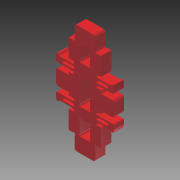
# Autodesk Inventor part: gantry7
Saved by Autodesk Inventor 2012 SP1 (Build 160190100, 190)
## iProperties
Created: 2011-10-14
Part Number: gantry7
Document SubType Name: Modeling
Designer: cramera
Density: 0.952 g/cm^3
Material: High Density Polyethylene
Mass: 48.8041 g
Surface Area: 201.117 cm^2
Volume: 51.2648 cm^3
Autodesk Inventor part; units mm, degrees
ref_plane "YZ Plane" through (0, 0, 0) normal (1, 0, 0) x (0, 1, 0)
ref_plane "XZ Plane" through (0, 0, 0) normal (0, 1, 0) x (-1, 0, 0)
ref_plane "XY Plane" through (0, 0, 0) normal (0, 0, 1) x (1, 0, 0)
derived "skeleton.ipt"
sketch "STOCK_12MM" plane through (0, 0, 0) normal (0, 0, 1) x (1, 0, 0)
  line L0 (457.2, 0) -> (914.4, 0)
  line L1 (914.4, 0) -> (914.4, 914.4)
  line L2 (914.4, 914.4) -> (457.2, 914.4)
  line L3 (457.2, 914.4) -> (457.2, 0)
  line L4 (0, 0) -> (457.2, 0)
  line L5 (457.2, 0) -> (457.2, 914.4)
  line L6 (457.2, 914.4) -> (0, 914.4)
  line L7 (0, 914.4) -> (0, 0)
  constraints: 16 end point
sketch "THROUGH-CUT" plane through (0, 0, 0) normal (0, 0, 1) x (1, 0, 0)
  arc A0 (280.404, 284.8782) -> (278.1589, 282.6331) centre (279.2814, 283.7556) ccw
  line L0 (278.1589, 282.6331) -> (278.1589, 255.1192)
  arc A1 (278.1589, 255.1192) -> (278.1589, 252.8742) centre (279.2814, 253.9967) ccw
  arc A2 (278.1589, 252.8742) -> (280.404, 252.8742) centre (279.2814, 253.9967) ccw
  line L1 (280.404, 252.8742) -> (288.2328, 252.8742)
  arc A3 (288.2328, 252.8742) -> (290.4779, 252.8742) centre (289.3554, 253.9967) ccw
  arc A4 (290.4779, 252.8742) -> (290.4779, 255.1192) centre (289.3554, 253.9967) ccw
  arc A5 (265.0779, 260.9387) -> (262.8328, 260.9387) centre (263.9554, 259.8161) ccw
  arc A6 (265.0779, 258.6936) -> (265.0779, 260.9387) centre (263.9554, 259.8161) ccw
  line L2 (265.0779, 258.6936) -> (265.0779, 257.6367)
  line L3 (265.0779, 257.6367) -> (269.8404, 257.6367)
  arc A7 (271.4279, 256.0492) -> (269.8404, 257.6367) centre (269.8404, 256.0492) ccw
  line L4 (271.4279, 256.0492) -> (271.4279, 255.9222)
  arc A8 (269.8404, 254.3347) -> (271.4279, 255.9222) centre (269.8404, 255.9222) ccw
  line L5 (269.8404, 254.3347) -> (265.0779, 254.3347)
  line L6 (265.0779, 254.3347) -> (251.4254, 254.3347)
  arc A9 (251.4254, 254.3347) -> (249.8379, 252.7494) centre (251.4254, 252.7472) ccw
  line L7 (249.8379, 252.7494) -> (249.8379, 249.0442)
  line L8 (249.8379, 249.0442) -> (250.66, 245.4447)
  line L9 (250.66, 245.4447) -> (252.3779, 245.4447)
  line L10 (252.3779, 245.4447) -> (253.6479, 246.9687)
  line L11 (253.6479, 246.9687) -> (256.2752, 246.9687)
  line L12 (256.2752, 246.9687) -> (265.0779, 246.9687)
  line L13 (265.0779, 246.9687) -> (269.8404, 246.9687)
  arc A10 (271.4279, 245.3812) -> (269.8404, 246.9687) centre (269.8404, 245.3812) ccw
  line L14 (271.4279, 245.3812) -> (271.4279, 245.2542)
  arc A11 (269.8404, 243.6667) -> (271.4279, 245.2542) centre (269.8404, 245.2542) ccw
  line L15 (269.8404, 243.6667) -> (265.0779, 243.6667)
  line L16 (265.0779, 243.6667) -> (265.0779, 222.2037)
  line L17 (265.0779, 222.2037) -> (269.8813, 222.2037)
  arc A12 (272.1264, 222.2037) -> (269.8813, 222.2037) centre (271.0039, 221.0811) ccw
  arc A13 (272.1264, 219.9586) -> (272.1264, 222.2037) centre (271.0039, 221.0811) ccw
  line L18 (272.1264, 219.9586) -> (272.1264, 206.3287)
  line L19 (272.1264, 206.3287) -> (273.7139, 204.7412)
  line L20 (273.7139, 204.7412) -> (294.9229, 204.7412)
  line L21 (294.9229, 204.7412) -> (296.5104, 206.3287)
  line L22 (296.5104, 206.3287) -> (296.5104, 219.9586)
  arc A14 (296.5104, 222.2037) -> (296.5104, 219.9586) centre (297.6329, 221.0811) ccw
  arc A15 (298.7555, 222.2037) -> (296.5104, 222.2037) centre (297.6329, 221.0811) ccw
  line L23 (298.7555, 222.2037) -> (303.5589, 222.2037)
  line L24 (303.5589, 222.2037) -> (303.5589, 243.6667)
  line L25 (303.5589, 243.6667) -> (298.7964, 243.6667)
  arc A16 (297.2089, 245.2542) -> (298.7964, 243.6667) centre (298.7964, 245.2542) ccw
  line L26 (297.2089, 245.2542) -> (297.2089, 245.3812)
  arc A17 (298.7964, 246.9687) -> (297.2089, 245.3812) centre (298.7964, 245.3812) ccw
  line L27 (298.7964, 246.9687) -> (303.5589, 246.9687)
  line L28 (303.5589, 246.9687) -> (312.3616, 246.9687)
  line L29 (312.3616, 246.9687) -> (314.9889, 246.9687)
  line L30 (314.9889, 246.9687) -> (316.2589, 245.4447)
  line L31 (316.2589, 245.4447) -> (317.9768, 245.4447)
  line L32 (317.9768, 245.4447) -> (318.7989, 249.0442)
  line L33 (318.7989, 249.0442) -> (318.7989, 252.7494)
  arc A18 (318.7989, 252.7494) -> (317.2114, 254.3347) centre (317.2114, 252.7472) ccw
  line L34 (317.2114, 254.3347) -> (303.5589, 254.3347)
  line L35 (303.5589, 254.3347) -> (298.7964, 254.3347)
  arc A19 (297.2089, 255.9222) -> (298.7964, 254.3347) centre (298.7964, 255.9222) ccw
  line L36 (297.2089, 255.9222) -> (297.2089, 256.0492)
  arc A20 (298.7964, 257.6367) -> (297.2089, 256.0492) centre (298.7964, 256.0492) ccw
  line L37 (298.7964, 257.6367) -> (303.5589, 257.6367)
  line L38 (303.5589, 257.6367) -> (303.5589, 258.6936)
  arc A21 (303.5589, 260.9387) -> (303.5589, 258.6936) centre (304.6814, 259.8161) ccw
  arc A22 (305.804, 260.9387) -> (303.5589, 260.9387) centre (304.6814, 259.8161) ccw
  line L39 (305.804, 260.9387) -> (317.2114, 260.9387)
  line L40 (317.2114, 260.9387) -> (318.7989, 262.5262)
  line L41 (318.7989, 262.5262) -> (318.7989, 277.1312)
  line L42 (318.7989, 277.1312) -> (317.2114, 278.7187)
  line L43 (317.2114, 278.7187) -> (305.804, 278.7187)
  arc A23 (303.5589, 280.9637) -> (305.804, 278.7187) centre (304.6814, 279.8412) ccw
  line L44 (303.5589, 280.9637) -> (303.5589, 282.0207)
  line L45 (303.5589, 282.0207) -> (298.7964, 282.0207)
  arc A24 (297.2089, 283.6082) -> (298.7964, 282.0207) centre (298.7964, 283.6082) ccw
  line L46 (297.2089, 283.6082) -> (297.2089, 283.7352)
  arc A25 (298.7964, 285.3227) -> (297.2089, 283.7352) centre (298.7964, 283.7352) ccw
  line L47 (298.7964, 285.3227) -> (303.5589, 285.3227)
  line L48 (303.5589, 285.3227) -> (317.2114, 285.3227)
  arc A26 (317.2114, 285.3227) -> (318.7989, 286.908) centre (317.2114, 286.9102) ccw
  line L49 (318.7989, 286.908) -> (318.7989, 290.6131)
  line L50 (318.7989, 290.6131) -> (317.9768, 294.2127)
  line L51 (317.9768, 294.2127) -> (316.2589, 294.2127)
  line L52 (316.2589, 294.2127) -> (314.9889, 292.6887)
  line L53 (314.9889, 292.6887) -> (312.3616, 292.6887)
  line L54 (312.3616, 292.6887) -> (303.5589, 292.6887)
  line L55 (303.5589, 292.6887) -> (298.7964, 292.6887)
  arc A27 (297.2089, 294.2762) -> (298.7964, 292.6887) centre (298.7964, 294.2762) ccw
  line L56 (297.2089, 294.2762) -> (297.2089, 294.4032)
  arc A28 (298.7964, 295.9907) -> (297.2089, 294.4032) centre (298.7964, 294.4032) ccw
  line L57 (298.7964, 295.9907) -> (303.5589, 295.9907)
  line L58 (303.5589, 295.9907) -> (303.5589, 317.4537)
  line L59 (303.5589, 317.4537) -> (298.7555, 317.4537)
  arc A29 (296.5104, 317.4537) -> (298.7555, 317.4537) centre (297.6329, 318.5762) ccw
  arc A30 (296.5104, 319.6987) -> (296.5104, 317.4537) centre (297.6329, 318.5762) ccw
  line L60 (296.5104, 319.6987) -> (296.5104, 333.3287)
  line L61 (296.5104, 333.3287) -> (294.9229, 334.9162)
  line L62 (294.9229, 334.9162) -> (273.7139, 334.9162)
  line L63 (273.7139, 334.9162) -> (272.1264, 333.3287)
  line L64 (272.1264, 333.3287) -> (272.1264, 319.6987)
  arc A31 (272.1264, 317.4537) -> (272.1264, 319.6987) centre (271.0039, 318.5762) ccw
  arc A32 (269.8813, 317.4537) -> (272.1264, 317.4537) centre (271.0039, 318.5762) ccw
  line L65 (269.8813, 317.4537) -> (265.0779, 317.4537)
  line L66 (265.0779, 317.4537) -> (265.0779, 295.9907)
  line L67 (265.0779, 295.9907) -> (269.8404, 295.9907)
  arc A33 (271.4279, 294.4032) -> (269.8404, 295.9907) centre (269.8404, 294.4032) ccw
  line L68 (271.4279, 294.4032) -> (271.4279, 294.2762)
  arc A34 (269.8404, 292.6887) -> (271.4279, 294.2762) centre (269.8404, 294.2762) ccw
  line L69 (269.8404, 292.6887) -> (265.0779, 292.6887)
  line L70 (265.0779, 292.6887) -> (256.2752, 292.6887)
  line L71 (256.2752, 292.6887) -> (253.6479, 292.6887)
  line L72 (253.6479, 292.6887) -> (252.3779, 294.2127)
  line L73 (252.3779, 294.2127) -> (250.66, 294.2127)
  line L74 (250.66, 294.2127) -> (249.8379, 290.6131)
  line L75 (249.8379, 290.6131) -> (249.8379, 286.908)
  arc A35 (249.8379, 286.908) -> (251.4254, 285.3227) centre (251.4254, 286.9102) ccw
  line L76 (251.4254, 285.3227) -> (265.0779, 285.3227)
  line L77 (265.0779, 285.3227) -> (269.8404, 285.3227)
  arc A36 (271.4279, 283.7352) -> (269.8404, 285.3227) centre (269.8404, 283.7352) ccw
  line L78 (271.4279, 283.7352) -> (271.4279, 283.6082)
  arc A37 (269.8404, 282.0207) -> (271.4279, 283.6082) centre (269.8404, 283.6082) ccw
  line L79 (269.8404, 282.0207) -> (265.0779, 282.0207)
  line L80 (265.0779, 282.0207) -> (265.0779, 280.9637)
  arc A38 (262.8328, 278.7187) -> (265.0779, 280.9637) centre (263.9554, 279.8412) ccw
  line L81 (262.8328, 278.7187) -> (251.4254, 278.7187)
  line L82 (251.4254, 278.7187) -> (249.8379, 277.1312)
  line L83 (249.8379, 277.1312) -> (249.8379, 262.5262)
  line L84 (249.8379, 262.5262) -> (251.4254, 260.9387)
  line L85 (251.4254, 260.9387) -> (262.8328, 260.9387)
  arc A39 (280.404, 317.4537) -> (278.1589, 317.4537) centre (279.2814, 316.3311) ccw
  arc A40 (278.1589, 317.4537) -> (278.1589, 315.2086) centre (279.2814, 316.3311) ccw
  line L86 (278.1589, 315.2086) -> (278.1589, 300.6487)
  arc A41 (278.1589, 300.6487) -> (278.1589, 298.4037) centre (279.2814, 299.5262) ccw
  arc A42 (278.1589, 298.4037) -> (280.404, 298.4037) centre (279.2814, 299.5262) ccw
  line L87 (280.404, 298.4037) -> (288.2328, 298.4037)
  arc A43 (288.2328, 298.4037) -> (290.4779, 300.6487) centre (289.3554, 299.5262) ccw
  line L88 (290.4779, 300.6487) -> (290.4779, 315.2086)
  arc A44 (290.4779, 315.2086) -> (290.4779, 317.4537) centre (289.3554, 316.3311) ccw
  arc A45 (290.4779, 317.4537) -> (288.2328, 317.4537) centre (289.3554, 316.3311) ccw
  line L89 (288.2328, 317.4537) -> (280.404, 317.4537)
  line L90 (278.1589, 239.0086) -> (278.1589, 224.4487)
  arc A46 (278.1589, 224.4487) -> (278.1589, 222.2037) centre (279.2814, 223.3262) ccw
  arc A47 (278.1589, 222.2037) -> (280.404, 222.2037) centre (279.2814, 223.3262) ccw
  line L91 (280.404, 222.2037) -> (288.2328, 222.2037)
  arc A48 (288.2328, 222.2037) -> (290.4779, 222.2037) centre (289.3554, 223.3262) ccw
  arc A49 (290.4779, 222.2037) -> (290.4779, 224.4487) centre (289.3554, 223.3262) ccw
  line L92 (290.4779, 224.4487) -> (290.4779, 239.0086)
  arc A50 (290.4779, 239.0086) -> (290.4779, 241.2537) centre (289.3554, 240.1311) ccw
  arc A51 (290.4779, 241.2537) -> (288.2328, 241.2537) centre (289.3554, 240.1311) ccw
  line L93 (288.2328, 241.2537) -> (280.404, 241.2537)
  arc A52 (280.404, 241.2537) -> (278.1589, 239.0086) centre (279.2814, 240.1311) ccw
  line L94 (290.4779, 255.1192) -> (290.4779, 282.6331)
  arc A53 (290.4779, 282.6331) -> (290.4779, 284.8782) centre (289.3554, 283.7556) ccw
  arc A54 (290.4779, 284.8782) -> (288.2328, 284.8782) centre (289.3554, 283.7556) ccw
  line L95 (288.2328, 284.8782) -> (280.404, 284.8782)
  arc A55 (258.312, 252.3027) -> (256.7245, 250.7152) centre (258.312, 250.7152) ccw
  line L96 (256.7245, 250.7152) -> (256.7245, 250.5882)
  arc A56 (256.7245, 250.5882) -> (258.312, 249.0007) centre (258.312, 250.5882) ccw
  line L97 (258.312, 249.0007) -> (269.8404, 249.0007)
  arc A57 (269.8404, 249.0007) -> (271.4279, 250.5882) centre (269.8404, 250.5882) ccw
  line L98 (271.4279, 250.5882) -> (271.4279, 250.7152)
  arc A58 (271.4279, 250.7152) -> (269.8404, 252.3027) centre (269.8404, 250.7152) ccw
  line L99 (269.8404, 252.3027) -> (258.312, 252.3027)
  arc A59 (269.8404, 287.3547) -> (271.4279, 288.9422) centre (269.8404, 288.9422) ccw
  line L100 (269.8404, 287.3547) -> (258.312, 287.3547)
  arc A60 (256.7245, 288.9422) -> (258.312, 287.3547) centre (258.312, 288.9422) ccw
  line L101 (256.7245, 288.9422) -> (256.7245, 289.0692)
  arc A61 (258.312, 290.6567) -> (256.7245, 289.0692) centre (258.312, 289.0692) ccw
  line L102 (258.312, 290.6567) -> (269.8404, 290.6567)
  arc A62 (271.4279, 289.0692) -> (269.8404, 290.6567) centre (269.8404, 289.0692) ccw
  line L103 (271.4279, 289.0692) -> (271.4279, 288.9422)
  arc A63 (297.2089, 288.9422) -> (298.7964, 287.3547) centre (298.7964, 288.9422) ccw
  line L104 (298.7964, 287.3547) -> (310.3248, 287.3547)
  arc A64 (310.3248, 287.3547) -> (311.9123, 288.9422) centre (310.3248, 288.9422) ccw
  line L105 (311.9123, 288.9422) -> (311.9123, 289.0692)
  arc A65 (311.9123, 289.0692) -> (310.3248, 290.6567) centre (310.3248, 289.0692) ccw
  line L106 (310.3248, 290.6567) -> (298.7964, 290.6567)
  arc A66 (298.7964, 290.6567) -> (297.2089, 289.0692) centre (298.7964, 289.0692) ccw
  line L107 (297.2089, 289.0692) -> (297.2089, 288.9422)
  arc A67 (297.2089, 250.5882) -> (298.7964, 249.0007) centre (298.7964, 250.5882) ccw
  line L108 (297.2089, 250.5882) -> (297.2089, 250.7152)
  arc A68 (298.7964, 252.3027) -> (297.2089, 250.7152) centre (298.7964, 250.7152) ccw
  line L109 (298.7964, 252.3027) -> (310.3248, 252.3027)
  arc A69 (311.9123, 250.7152) -> (310.3248, 252.3027) centre (310.3248, 250.7152) ccw
  line L110 (311.9123, 250.7152) -> (311.9123, 250.5882)
  arc A70 (310.3248, 249.0007) -> (311.9123, 250.5882) centre (310.3248, 250.5882) ccw
  line L111 (310.3248, 249.0007) -> (298.7964, 249.0007)
  constraints: 224 end point, 142 point on circle, 71 centre point
extrude "Extrusion1" add sketch "THROUGH-CUT" along normal blind 12
equation "\"d1\" = StockThickness"
equation "\"StockThickness\" = 12"
body "Solid1"
